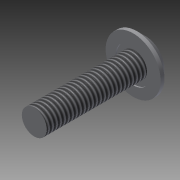
# Autodesk Inventor part: M5x20BlindScrew
Saved by Autodesk Inventor 2015 SP1 (Build 190203100, 203)
## iProperties
Category: Hardware
Created: 2013-12-08
Part Number: M5x20BlindScrew
Material: Stainless Steel
Document SubType Name: Modeling
Designer: Jack
Density: 8.08 g/cm^3
Appearance: Semi-Polished
Mass: 4.42636 g
Surface Area: 5.8331 cm^2
Volume: 0.547817 cm^3
Vendor: Misumi
Catalog Web Link: http://us.misumi-ec.com/vona2/detail/110300464310/
Stock Number: HTJ5
Author: Misumi
Title: Blind Screw 5mm
Autodesk Inventor part; units mm, degrees
ref_plane "YZ Plane" through (0, 0, 0) normal (1, 0, 0) x (0, 1, 0)
ref_plane "XZ Plane" through (0, 0, 0) normal (0, 1, 0) x (-1, 0, 0)
ref_plane "XY Plane" through (0, 0, 0) normal (0, 0, 1) x (1, 0, 0)
sketch "Sketch1" plane through (0, 0, 0) normal (0, 1, 0) x (-1, 0, 0)
  circle A0 centre (0, 0) radius 2.5
  dimension "d0" = 5
  constraints: 1 centre point, 1 coincident
  measures "d0" diameter of A0
extrude "Extrusion1" add sketch "Sketch1" along normal blind 20
sketch "Sketch2" plane through (0, 20, 0) normal (0, 1, 0) x (1, 0, 0)
  circle A0 centre (0, 0) radius 2.5 projected
  circle A1 centre (0, 0) radius 5.5
  dimension "d3" = 11
  constraints: 1 centre point, 1 coincident
  measures "d3" diameter of A1
extrude "Extrusion2" add sketch "Sketch2" along normal blind 2.25 contours A0 | A1
sketch "Sketch3" plane through (0, 22.25, 0) normal (0, 1, 0) x (1, 0, 0)
  circle A0 centre (0, 0) radius 5.5 projected
  line L0 (0, 2.217) -> (1.92, 1.1085)
  line L1 (1.92, 1.1085) -> (1.92, -1.1085)
  line L2 (1.92, -1.1085) -> (0, -2.217)
  line L3 (0, -2.217) -> (-1.92, -1.1085)
  line L4 (-1.92, -1.1085) -> (-1.92, 1.1085)
  line L5 (-1.92, 1.1085) -> (0, 2.217)
  dimension "d6" = 1.92
  constraints: 12 end point, 1 coincident, 1 vertical, 13 other
  measures "d6" distance from line of point (0, 0) L4
chamfer "Chamfer1" distance 1.75 angle 45 1 edges at (-5.5, 22.25, 0)
sketch "Sketch4" plane through (0, 20, 0) normal (0, -1, 0) x (1, 0, 0)
  circle A0 centre (0, 0) radius 5.5 projected
  circle A1 centre (0, 0) radius 2.5 projected
  circle A2 centre (0, 0) radius 3.5
  dimension "d10" = 7
  constraints: 1 centre point, 1 coincident
  measures "d10" diameter of A2
extrude "Extrusion3" add sketch "Sketch4" along normal blind 0.25 contours A0
extrude "Extrusion4" cut sketch "Sketch3" against normal blind 2 contours L0 L1 L2 L3 L4 L5
thread "Thread1" size "M5x0.8" class "6g" standard "ANSI Metric M Profile" full length
body "Solid1"
